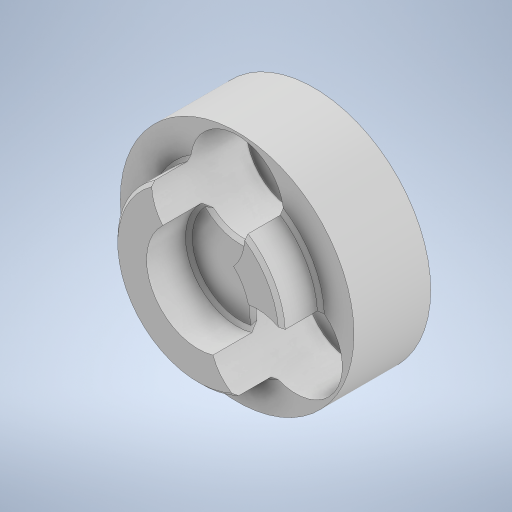
# Autodesk Inventor part: acc_motor_maghold
Saved by Autodesk Inventor 2023 (Build 270158000, 158)
## iProperties
Created: 2023-11-23
Part Number: acc_motor_maghold
Material: Generic
Document SubType Name: Modeling
Designer: aaron
Density: 1 g/cm^3
Appearance: Default
Author: aaron
Autodesk Inventor part; units mm, degrees
ref_plane "YZ Plane" through (0, 0, 0) normal (1, 0, 0) x (0, 1, 0)
ref_plane "XZ Plane" through (0, 0, 0) normal (0, 1, 0) x (-1, 0, 0)
ref_plane "XY Plane" through (0, 0, 0) normal (0, 0, 1) x (1, 0, 0)
sketch "Sketch1" plane through (0, 0, 0) normal (0, 0, 1) x (1, 0, 0)
  circle A0 centre (0, 0) radius 6.9
  line L0 (0, 0) -> (0, 9.7668)
  circle A1 centre (0, 0) radius 4
  circle A2 centre (0, 4) radius 1.5
  circle A3 centre (-3.4641, -2) radius 1.5
  circle A4 centre (3.4641, -2) radius 1.5
  dimension "d1" = 8
  dimension "d0" = 13.8
  dimension "d2" = 3
  dimension "d5" = 360
  constraints: 4 centre point, 2 coincident, 2 end point, 1 point on line, 1 vertical, 1 vertical alignment, 9 other
  measures "d0" diameter of A0
  measures "d2" diameter of A2
extrude "Extrusion1" add sketch "Sketch1" along normal blind 4.53 contours A0 | A2 A1 A4 A3 | A3 A1 | A1 A3
sketch "Sketch2" plane through (0, 0, 4.53) normal (0, 0, 1) x (1, 0, 0)
  circle A0 centre (0, 0) radius 4.95
  dimension "d9" = 9.9
  constraints: 1 centre point, 1 coincident
  measures "d9" diameter of A0
extrude "Extrusion2" add sketch "Sketch2" along normal blind 2.3
sketch "Sketch3" plane through (0, 0, 6.83) normal (0, 0, 1) x (1, 0, 0)
  circle A0 centre (0, 0) radius 3.05
  dimension "d12" = 6.1
  constraints: 1 centre point, 1 coincident
  measures "d12" diameter of A0
extrude "Extrusion3" cut sketch "Sketch3" against normal blind 2.5
sketch "Sketch4" plane through (0, 0, 6.83) normal (0, 0, 1) x (1, 0, 0)
  arc A0 (1.2803, 4.7816) -> (-1.2803, 4.7816) centre (0, 4) ccw projected
  circle A1 centre (0, 4) radius 2.75
  circle A2 centre (-3.4641, -2) radius 2.75
  circle A3 centre (3.4641, -2) radius 2.75
  point P0 (0, 0)
  dimension "d15" = 5.5
  dimension "d18" = 360
  constraints: 3 centre point, 1 coincident, 7 other
  measures "d15" diameter of A1
extrude "Extrusion4" cut sketch "Sketch4" against normal blind 5.6 contours A1 | A3
chamfer "Chamfer1" distance 0.2 angle 45 2 edges at (2.6414, 1.525, 4.33) (-2.6414, -1.525, 4.33)
chamfer "Chamfer2" distance 0.2 angle 45 2 edges at (4.2868, 2.475, 6.83) (-4.2868, -2.475, 6.83)
chamfer "Chamfer3" distance 0.2 angle 45 4 edges at (-1.5, 4, 1.23) (0, 1.25, 4.33) (1.0825, -0.625, 4.33) (1.9641, -2, 1.23)
chamfer "Chamfer4" distance 0.2 angle 45 2 edges at (4.2868, 2.475, 4.53) (-4.2868, -2.475, 4.53)
body "Solid1"
